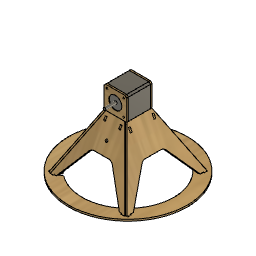
stepper stand v6 (Autodesk Fusion 360 design; units mm, degrees)
Autodesk Fusion 360 part; units mm, degrees
(part 1 of 2)
sketch "Sketch1" plane through (0, 0, 0) normal (0, 1, 0) x (1, 0, 0) in component "stepper"
  circle A0 centre (0, 0) radius 2.5
  circle A1 centre (0, 0) radius 12
  line L0 (21, 21) -> (-21, 21)
  line L1 (-21, 21) -> (-21, -21)
  line L2 (-21, -21) -> (21, -21)
  line L3 (21, -21) -> (21, 21)
  line L4 (21, 21) -> (-21, -21) construction
  line L5 (-21, 21) -> (21, -21) construction
  line L6 (-15.5, -15.5) -> (15.5, -15.5) construction
  line L7 (15.5, -15.5) -> (15.5, 15.5) construction
  line L8 (15.5, 15.5) -> (-15.5, 15.5) construction
  line L9 (-15.5, 15.5) -> (-15.5, -15.5) construction
  line L10 (-15.5, -15.5) -> (15.5, 15.5) construction
  line L11 (15.5, -15.5) -> (-15.5, 15.5) construction
  circle A2 centre (15.5, -15.5) radius 1.5
  circle A3 centre (-15.5, -15.5) radius 1.5
  circle A4 centre (-15.5, 15.5) radius 1.5
  circle A5 centre (15.5, 15.5) radius 1.5
  dimension "d1" = 5
  dimension "d2" = 24
  dimension "d3" = 42
  dimension "d4" = 42
  dimension "d5" = 31
  dimension "d6" = 31
  dimension "d7" = 3
  dimension "d8" = 3
  dimension "d9" = 3
  dimension "d10" = 3
  constraint coincident A0.centre A1.centre
  constraint concentric A0 A1
  constraint horizontal L0
  constraint perpendicular L0 L1
  constraint parallel L0 L2
  constraint parallel L1 L3
  constraint coincident L4 A0.centre
  constraint coincident L5 A0.centre
  constraint horizontal L6
  constraint perpendicular L6 L7
  constraint parallel L6 L8
  constraint parallel L7 L9
  constraint coincident L10 A0.centre
  constraint coincident L11 A0.centre
  constraint coincident L6.end L7.start
  constraint coincident L6.start L9.end
  constraint coincident L8.end L9.start
  constraint coincident L7.end L8.start
  measures "d1" diameter of A0
  measures "d2" diameter of A1
  measures "d3" distance of L1.end L2.end
  measures "d4" distance of L0.end L1.end
  measures "d5" distance of L7.end L8.end
  measures "d6" distance of L6.end L7.end
  measures "d7" diameter of A2
  measures "d8" diameter of A3
  measures "d9" diameter of A4
  measures "d10" diameter of A5
extrude "Extrude1" add sketch "Sketch1" against normal blind 41 from surface at 20.5 contours A0 | A1 | L0 L1 L2 L3 | A2 | A3 | A4 | A5 makes body 1 in component "stepper"
extrude "Extrude2" add sketch "Sketch1" against normal blind 2 from surface at -20.5 contours A0 | A1 bodies 1 in component "stepper"
extrude "Extrude3" add sketch "Sketch1" against normal blind 21 from surface at -22.5 contours A0 bodies 1 in component "stepper"
extrude "Extrude4" cut sketch "Sketch1" along normal blind 5 from surface at -20.5 contours A2 | A3 | A4 | A5 bodies 1 in component "stepper"
sketch "Sketch1 (2)" plane through (0, 0, 0) normal (0, 1, 0) x (1, 0, 0) in component "front plate"
  circle A0 centre (15.5, -15.5) radius 1.5
  circle A1 centre (15.5, 15.5) radius 1.5
  circle A2 centre (-15.5, -15.5) radius 1.5
  circle A3 centre (-15.5, 15.5) radius 1.5
  circle A4 centre (0, 0) radius 12
  line L0 (21, 21) -> (21, -21)
  line L1 (21, -21) -> (-21, -21)
  line L2 (-21, -21) -> (-21, 21)
  line L3 (-21, 21) -> (21, 21)
  line L4 (0, 21) -> (0, 121) construction
  line L5 (-142.4653, 121) -> (140, 121) construction
  line L6 (21, 21) -> (71.9525, 121)
  line L7 (21, 21) -> (155.3334, 21) construction
  line L8 (-21, 21) -> (-71.9525, 121)
  line L9 (13.9709, 71) -> (-46.4763, 71)
  line L10 (-17.633, 21) -> (-68.5856, 121)
  line L11 (17.633, 21) -> (68.5856, 121)
  line L12 (-21, 21) -> (-18.327, 22.362)
  line L13 (21, 21) -> (18.327, 22.362)
  line L14 (-25.2759, 36) -> (25.2759, 36)
  line L15 (68.5856, 121) -> (58.5856, 121)
  line L16 (58.5856, 121) -> (21.7954, 74.7728)
  arc A5 (13.9709, 71) -> (21.7954, 74.7728) centre (13.9709, 81) ccw
  line L17 (-68.5856, 121) -> (-58.5856, 121)
  line L18 (-58.5856, 121) -> (-21.7954, 74.7728)
  arc A6 (-21.7954, 74.7728) -> (-13.9709, 71) centre (-13.9709, 81) ccw
  line L19 (25.2759, 36) -> (27.9489, 34.638)
  line L20 (24.317, 27.51) -> (21.644, 28.8719)
  line L21 (-25.2759, 36) -> (-27.9489, 34.638)
  line L22 (-24.317, 27.51) -> (-21.644, 28.8719)
  line L23 (12.5, 21) -> (12.5, 36)
  line L24 (15.5, 21) -> (15.5, 36)
  line L25 (12.5, 28.5) -> (15.5, 28.5)
  line L26 (-12.5, 21) -> (-12.5, 36)
  line L27 (-15.5, 21) -> (-15.5, 36)
  line L28 (-12.5, 28.5) -> (-15.5, 28.5)
  dimension "d23" = 100
  dimension "d24" = 63
  dimension "d25" = 50
  dimension "d28" = 3
  dimension "d29" = 3
  dimension "d30" = 15
  dimension "d31" = 10
  dimension "d32" = 10
  dimension "d33" = 8
  dimension "d34" = 12.5
  dimension "d35" = 3
  constraint midpoint L3 L4.start
  constraint perpendicular L3 L4
  constraint perpendicular L4 L5
  constraint horizontal L7
  constraint coincident L0.start L3.end
  constraint coincident L5 L6.end
  constraint symmetric L4 L0.start L2.end
  constraint symmetric L4 L6.end L8.end
  constraint coincident L4.end L5
  constraint coincident L8 L9.end
  constraint horizontal L9
  constraint parallel L8 L10
  constraint coincident L3 L10.start
  constraint parallel L6 L11
  constraint coincident L3 L11.start
  constraint coincident L2.end L3.start
  constraint coincident L10 L12.end
  constraint perpendicular L10 L12
  constraint coincident L11 L13.end
  constraint perpendicular L11 L13
  constraint coincident L10 L14.start
  constraint coincident L11 L14.end
  constraint horizontal L14
  constraint coincident L5 L10.end
  constraint coincident L5 L11.end
  constraint coincident L5 L15.end
  constraint coincident L2.end L16
  constraint tangent L16 A5
  constraint tangent L9 A5
  constraint symmetric L4 L11.end L10.end
  constraint symmetric L4 L15.end L17.end
  constraint symmetric L4 L16.end L18.end
  constraint symmetric L4 L9.start A6.end
  constraint symmetric L4 A5 A6
  constraint coincident L6 L19.end
  constraint perpendicular L6 L19
  constraint coincident L6 L20.start
  constraint coincident L11 L20.end
  constraint perpendicular L11 L20
  constraint symmetric L4 L14.end L14.start
  constraint symmetric L4 L19.end L21.end
  constraint symmetric L4 L20.start L22.start
  constraint symmetric L4 L20.end L22.end
  constraint coincident L3 L23.start
  constraint coincident L14 L23.end
  constraint perpendicular L14 L23
  constraint coincident L3 L24.start
  constraint coincident L14 L24.end
  constraint perpendicular L14 L24
  constraint midpoint L23 L25.start
  constraint midpoint L24 L25.end
  constraint symmetric L4 L23.start L26.start
  constraint symmetric L4 L23.end L26.end
  constraint symmetric L4 L24.start L27.start
  constraint symmetric L4 L24.end L27.end
  constraint symmetric L4 L25.start L28.start
  constraint symmetric L4 L25.end L28.end
  measures "d23" distance of L4.start L4.end
  measures "d24" angle of L6 L7
  measures "d25" distance of L3 L9
  measures "d28" distance of L0.start L13.end
  measures "d29" distance of L2.end L12.end
  measures "d30" distance of L3 L14
  measures "d31" distance of L11.end L15.end
  measures "d32" radius of A5
  measures "d33" distance of L19 L20
  measures "d34" distance of L4 L23
  measures "d35" distance of L23 L24
extrude "Extrude1'" add sketch "Sketch1 (2)" against normal blind 3 from surface at -20.5 separate body contours L0 L1 L2 L3 | L3 L11 L14 L24 | L6 L11 L19 L20 | L3 L23 L24 L25 | L3 L14 L23 L26 | L3 L10 L14 L27 | L8 L10 L21 L22 | L3 L26 L27 L28 makes body 2 in component "front plate"
extrude "Extrude2'" add sketch "Sketch1 (2)" along normal blind 3 from surface at 20.5 separate body contours A0 | A1 | A2 | A3 | A4 | L0 L1 L2 L3 | L3 L11 L14 L24 | L6 L11 L19 L20 | L3 L23 L24 L25 | L3 L14 L23 L26 | L3 L10 L14 L27 | L8 L10 L21 L22 | L3 L26 L27 L28 makes body 3 in component "front plate"
sketch "Sketch1 (3)" plane through (0, 0, 0) normal (1, 0, 0) x (0, 1, 0) in component "side plate"
  line L0 (20.5, -21) -> (20.5, 21)
  line L1 (20.5, 21) -> (-20.5, 21)
  line L2 (-20.5, 21) -> (-20.5, -21)
  line L3 (-20.5, -21) -> (20.5, -21)
  line L4 (20.5, 21) -> (20.5, -21)
  line L5 (20.5, -21) -> (23.5, -21)
  line L6 (23.5, -21) -> (23.5, 21)
  line L7 (23.5, 21) -> (20.5, 21)
  line L8 (-20.5, -21) -> (-20.5, 21)
  line L9 (-20.5, 21) -> (-23.5, 21)
  line L10 (-23.5, 21) -> (-23.5, -21)
  line L11 (-23.5, -21) -> (-20.5, -21)
  line L12 (-20.5, -36) -> (-20.5, -28.5)
  line L13 (-20.5, -28.5) -> (-23.5, -28.5)
  line L14 (-23.5, -28.5) -> (-23.5, -36)
  line L15 (-23.5, -36) -> (-20.5, -36)
  line L16 (20.5, -28.5) -> (20.5, -36)
  line L17 (20.5, -36) -> (23.5, -36)
  line L18 (23.5, -36) -> (23.5, -28.5)
  line L19 (23.5, -28.5) -> (20.5, -28.5)
  line L20 (-165.7609, -120.8985) -> (170, -120.8985) construction
  line L21 (0, 0) -> (0, -121) construction
  line L22 (23.5, -21) -> (74.4008, -120.8985)
  line L23 (23.5, -21) -> (135.2326, -21) construction
  line L24 (-23.5, -21) -> (-74.4008, -120.8985)
  line L25 (-31.1429, -36) -> (31.1429, -36)
  line L26 (20.133, -21) -> (71.0338, -120.8985)
  line L27 (23.5, -28.5) -> (26.5338, -26.9542)
  line L28 (23.5, -36) -> (29.5676, -32.9084)
  line L29 (-20.133, -21) -> (-71.0338, -120.8985)
  line L30 (-23.5, -36) -> (-29.5676, -32.9084)
  line L31 (-23.5, -28.5) -> (-26.5338, -26.9542)
  line L32 (-20.5, 21) -> (-20.5, -21)
  line L33 (20.5, 21) -> (20.5, -21)
  line L34 (-20.5, -28.5) -> (-20.5, -21)
  line L35 (20.5, -28.5) -> (20.5, -21)
  point P0 (0, -121)
  dimension "d42" = 63
  dimension "d43" = 3
  constraint horizontal L20
  constraint coincident L21.start origin
  constraint coincident P0 L21.end
  constraint horizontal L23
  constraint coincident L5.end L6.start
  constraint coincident L20 L22.end
  constraint symmetric L21 L5.end L10.end
  constraint symmetric L21 L22.end L24.end
  constraint coincident L24 L25.start
  constraint coincident L22 L25.end
  constraint horizontal L25
  constraint collinear L17 L25
  constraint coincident L3 L26.start
  constraint coincident L20 L26.end
  constraint parallel L22 L26
  constraint coincident L18.end L19.start
  constraint coincident L22 L27.end
  constraint perpendicular L22 L27
  constraint coincident L17.end L18.start
  constraint coincident L22 L28.end
  constraint perpendicular L22 L28
  constraint symmetric L21 L26.start L29.start
  constraint symmetric L21 L26.end L29.end
  constraint symmetric L21 L18.end L13.end
  constraint symmetric L21 L27.end L31.end
  constraint symmetric L21 L17.end L14.end
  constraint symmetric L21 L28.end L30.end
  constraint coincident L12.end L13.start
  constraint coincident L2.end L3.start
  constraint coincident L16.start L19.end
  constraint coincident L0.start L3.end
  measures "d42" angle of L22 L23
  measures "d43" distance of L22 L26
extrude "Extrude1''" add sketch "Sketch1 (3)" along normal blind 3 from surface at 12.5 separate body contours L3 L12 L16 L25 L26 L29 L34 L35 | L22 L26 L27 L28 | L18 L26 L27 L28 | L16 L17 L18 L19 L25 | L25 L26 L28 | L14 L29 L30 L31 | L24 L29 L30 L31 | L12 L13 L14 L15 L25 | L25 L29 L30 makes body 4 in component "side plate"
mirror "Mirror1" about plane through (0, 0, 0) normal (1, 0, 0) of bodies 4 makes body 5 in component "side plate"
sketch "Sketch2" plane through (0, 0, 0) normal (0, 1, 0) x (1, 0, 0) in component "front face"
  line L0 (58.5856, 121) -> (21.7954, 74.7728)
  arc A0 (13.9709, 71) -> (21.7954, 74.7728) centre (13.9709, 81) ccw
  arc A1 (-21.7954, 74.7728) -> (-13.9709, 71) centre (-13.9709, 81) ccw
  line L1 (13.9709, 71) -> (-46.4763, 71)
  line L2 (-58.5856, 121) -> (-21.7954, 74.7728)
  line L3 (-68.5856, 121) -> (-58.5856, 121)
  line L4 (-17.633, 21) -> (-68.5856, 121)
  line L5 (-21, 21) -> (21, 21)
  line L6 (17.633, 21) -> (68.5856, 121)
  line L7 (68.5856, 121) -> (58.5856, 121)
  line L8 (68.5856, 121) -> (62.5856, 121)
  line L9 (62.5856, 121) -> (62.5856, 124)
  line L10 (62.5856, 124) -> (68.5856, 124)
  line L11 (68.5856, 124) -> (68.5856, 121)
  line L12 (0, 21) -> (0, 121)
  line L13 (-62.5856, 121) -> (-62.5856, 124)
  line L14 (-68.5856, 121) -> (-62.5856, 121)
  line L15 (-68.5856, 124) -> (-68.5856, 121)
  line L16 (-62.5856, 124) -> (-68.5856, 124)
  point P0 (-68.5856, 121)
  point P1 (-68.5856, 121)
  dimension "d53" = 6
  dimension "d54" = 3
  constraint horizontal L8
  constraint vertical L9
  constraint horizontal L10
  constraint vertical L11
  constraint coincident L6.end L7.start
  constraint symmetric L6.end L12 P1
  constraint symmetric L8.end L12 L13.start
  constraint symmetric L9.end L12 L13.end
  constraint symmetric L10.end L12 L15.start
  measures "d53" distance of L6.end L8.end
  measures "d54" distance of L6.end L10.end
extrude "Extrude1'''" add sketch "Sketch2" along normal blind -200 and the other way blind -200 separate body makes body 6 in component "front face"
ref_plane "WorkPlane1" through (-14, -28.0507, -29.9313) normal (0, -0.891007, 0.45399) x (0, -0.45399, -0.891007) in component "front face"
split "Split1" by plane through (-14, -28.0507, -29.9313) normal (0, -0.891007, 0.45399) bodies 6 makes body 7 at (34.6172, -99.3175, -54.3333) in component "front face"
sketch "Sketch3" plane through (0, -10.1618, 5.1777) normal (0, -0.891007, 0.45399) x (1, 0, 0) in component "front face"
  line L0 (68.5856, -141.6125) -> (17.633, -29.3799)
  line L1 (17.633, -29.3799) -> (-17.633, -29.3799)
  line L2 (-17.633, -29.3799) -> (-68.5856, -141.6125)
  line L3 (-62.5856, -141.6125) -> (-58.5856, -141.6125)
  line L4 (-58.5856, -141.6125) -> (-21.7954, -89.7306)
  ellipse E0 centre (-13.9709, -96.7195) end of major axis (-13.9709, -85.4962) minor radius 10 (-13.9709, -85.4962) -> (-21.7954, -89.7306) ccw
  line L5 (-13.9709, -85.4962) -> (13.9709, -85.4962)
  ellipse E1 centre (13.9709, -96.7195) end of major axis (13.9709, -85.4962) minor radius 10 (21.7954, -89.7306) -> (13.9709, -85.4962) ccw
  line L6 (21.7954, -89.7306) -> (58.5856, -141.6125)
  line L7 (58.5856, -141.6125) -> (62.5856, -141.6125)
  line L8 (-17.633, -29.3799) -> (-68.3511, -141.0961)
  line L9 (-68.3511, -141.0961) -> (-60.9204, -141.0961)
  line L10 (-60.9204, -141.0961) -> (-24.729, -90.0586)
  ellipse E2 centre (-13.9709, -96.7195) end of major axis (-13.7968, -84.6799) minor radius 12.8971 (-13.9966, -84.6784) -> (-24.729, -90.0586) ccw
  line L11 (-13.9966, -84.6784) -> (13.8126, -84.6784)
  ellipse E3 centre (13.9709, -96.7195) end of major axis (13.5291, -84.6836) minor radius 9.6471 (21.1526, -88.8241) -> (13.8126, -84.6784) ccw
  line L12 (21.1526, -88.8241) -> (58.5856, -141.6125)
  line L13 (58.5856, -141.6125) -> (68.5856, -141.6125)
  line L14 (68.5856, -141.6125) -> (17.633, -29.3799)
  line L15 (17.633, -29.3799) -> (-17.633, -29.3799)
  line L16 (-68.5856, -144.9795) -> (-62.5856, -144.9795)
  line L17 (-62.5856, -144.9795) -> (-62.5856, -141.6125)
  line L18 (62.5856, -141.6125) -> (62.5856, -144.9795)
  line L19 (62.5856, -144.9795) -> (68.5856, -144.9795)
  line L20 (68.5856, -144.9795) -> (68.5856, -141.6125)
  line L21 (-68.5856, -141.6125) -> (-68.5856, -144.9795)
  line L22 (-12.5, -42.745) -> (-12.5, -36.0625)
  line L23 (-12.5, -36.0625) -> (-15.5, -36.0625)
  line L24 (-15.5, -36.0625) -> (-15.5, -42.745)
  line L25 (-15.5, -42.745) -> (-12.5, -42.745)
  line L26 (12.5, -36.0625) -> (12.5, -42.745)
  line L27 (12.5, -42.745) -> (15.5, -42.745)
  line L28 (15.5, -42.745) -> (15.5, -36.0625)
  line L29 (15.5, -36.0625) -> (12.5, -36.0625)
  circle A0 centre (0, -65) radius 2.25
  dimension "d55" = 4.5
  constraint parallel L2 L8
  constraint parallel L3 L9
  constraint parallel L4 L10
  constraint concentric E0 E2
  constraint parallel L5 L11
  constraint concentric E1 E3
  constraint parallel L6 L12
  constraint parallel L7 L13
  constraint parallel L0 L14
  constraint parallel L1 L15
  constraint tangent L10 E2
  constraint tangent E2 L11
  constraint tangent E3 L12
  constraint tangent L11 E3
  measures "d55" diameter of A0
extrude "Extrude2''" add sketch "Sketch3" against normal blind 3 separate body makes body 8 in component "front face"
draft "Draft1" angle -63 neutral plane through (0, -10.1618, 5.1777) pull (0, -0.891007, 0.45399) 1 faces at (5.8777, -22.609, -21.454) on bodies 8 in component "front face"
ref_plane "WorkPlane2" through (14, 28.0507, -29.9313) normal (0, 0.891007, 0.45399) x (0, -0.45399, 0.891007) in component "front face"
split "Split2" by plane through (14, 28.0507, -29.9313) normal (0, 0.891007, 0.45399) bodies 6 makes body 9 at (34.6172, 99.3175, -54.3333) in component "front face"
sketch "Sketch4" plane through (0, 10.1618, 5.1777) normal (0, 0.891007, 0.45399) x (-1, 0, 0) in component "front face"
  line L0 (-62.5856, -141.6125) -> (-58.5856, -141.6125)
  line L1 (-58.5856, -141.6125) -> (-21.7954, -89.7306)
  ellipse E0 centre (-13.9709, -96.7195) end of major axis (-13.9709, -85.4962) minor radius 10 (-13.9709, -85.4962) -> (-21.7954, -89.7306) ccw
  line L2 (-13.9709, -85.4962) -> (13.9709, -85.4962)
  ellipse E1 centre (13.9709, -96.7195) end of major axis (13.9709, -85.4962) minor radius 10 (21.7954, -89.7306) -> (13.9709, -85.4962) ccw
  line L3 (21.7954, -89.7306) -> (58.5856, -141.6125)
  line L4 (58.5856, -141.6125) -> (62.5856, -141.6125)
  line L5 (62.5856, -141.6125) -> (62.5856, -144.9795)
  line L6 (62.5856, -144.9795) -> (68.5856, -144.9795)
  line L7 (68.5856, -144.9795) -> (68.5856, -141.6125)
  line L8 (68.5856, -141.6125) -> (17.633, -29.3799)
  line L9 (17.633, -29.3799) -> (-17.633, -29.3799)
  line L10 (-17.633, -29.3799) -> (-68.5856, -141.6125)
  line L11 (-68.5856, -141.6125) -> (-68.5856, -144.9795)
  line L12 (-68.5856, -144.9795) -> (-62.5856, -144.9795)
  line L13 (-62.5856, -144.9795) -> (-62.5856, -141.6125)
  line L14 (-17.633, -29.3799) -> (-68.5856, -141.6125)
  line L15 (-68.5856, -141.6125) -> (-68.5856, -144.9795)
  line L16 (-68.5856, -144.9795) -> (-62.5856, -144.9795)
  line L17 (-62.5856, -144.9795) -> (-62.5856, -141.6125)
  line L18 (-62.5856, -141.6125) -> (-58.5856, -141.6125)
  line L19 (-58.5856, -141.6125) -> (-21.7954, -89.7306)
  ellipse E2 centre (-13.9709, -96.7195) end of major axis (-13.9709, -85.4962) minor radius 10 (-13.9709, -85.4962) -> (-21.7954, -89.7306) ccw
  line L20 (-13.9709, -85.4962) -> (13.9709, -85.4962)
  ellipse E3 centre (13.9709, -96.7195) end of major axis (13.9709, -85.4962) minor radius 10 (21.7954, -89.7306) -> (13.9709, -85.4962) ccw
  line L21 (21.7954, -89.7306) -> (58.5856, -141.6125)
  line L22 (58.5856, -141.6125) -> (62.5856, -141.6125)
  line L23 (62.5856, -141.6125) -> (62.5856, -144.9795)
  line L24 (62.5856, -144.9795) -> (68.5856, -144.9795)
  line L25 (68.5856, -144.9795) -> (68.5856, -141.6125)
  line L26 (68.5856, -141.6125) -> (17.633, -29.3799)
  line L27 (17.633, -29.3799) -> (-17.633, -29.3799)
  line L28 (-12.5, -42.745) -> (-12.5, -36.0625)
  line L29 (-12.5, -36.0625) -> (-15.5, -36.0625)
  line L30 (-15.5, -36.0625) -> (-15.5, -42.745)
  line L31 (-15.5, -42.745) -> (-12.5, -42.745)
  line L32 (12.5, -36.0625) -> (12.5, -42.745)
  line L33 (12.5, -42.745) -> (15.5, -42.745)
  line L34 (15.5, -42.745) -> (15.5, -36.0625)
  line L35 (15.5, -36.0625) -> (12.5, -36.0625)
  line L36 (0, -29.3799) -> (0, -121.839) construction
  circle A0 centre (0, -70.4962) radius 5.5
  circle A1 centre (0, -55.4962) radius 3
  dimension "d63" = 0
  dimension "d64" = 11
  dimension "d65" = 15
  dimension "d66" = 6
  dimension "d67" = 30
  constraint midpoint L27 L36.start
  constraint perpendicular L9 L36
  constraint coincident L36 A0.centre
  constraint coincident L36 A1.centre
  measures "d64" diameter of A0
  measures "d65" distance of L20 A0.centre
  measures "d66" diameter of A1
  measures "d67" distance of L20 A1.centre
extrude "Extrude3'" add sketch "Sketch4" against normal blind 3 separate body makes body 10 in component "front face"
draft "Draft2" angle -63 neutral plane through (0, 10.1618, 5.1777) pull (0, 0.891007, 0.45399) 1 faces at (-5.8777, 22.609, -21.454) on bodies 10 in component "front face"
ref_plane "WorkPlane1" through (0, 0, -121) normal (0, 0, 1) x (1, 0, 0) in component "sides"
sketch "Sketch3 (2)" plane through (0, 0, 0) normal (1, 0, 0) x (0, 1, 0) in component "sides"
  line L0 (74.4525, -121) -> (23.5, -21)
  line L1 (-23.5, -21) -> (-74.4525, -121)
  line L2 (35.783, -121) -> (1.2339, -121)
  line L3 (-23.5, -21) -> (23.5, -21)
  line L4 (-62.4525, -121) -> (-22.4689, -74.4817)
  line L5 (0, -71) -> (-14.8852, -71)
  arc A0 (-14.8852, -71) -> (-22.4689, -74.4817) centre (-14.8852, -81) ccw
  line L6 (-62.4525, -121) -> (23.5, -21) construction
  line L7 (0, -21) -> (0, -121) construction
  line L8 (0, -21) -> (0, -121)
  line L9 (-62.4525, -121) -> (-74.4525, -121)
  line L10 (-74.4525, -121) -> (-68.4525, -121)
  line L11 (-68.4525, -121) -> (-68.4525, -124)
  line L12 (-68.4525, -124) -> (-74.4525, -124)
  line L13 (-74.4525, -124) -> (-74.4525, -121)
  line L14 (62.4525, -121) -> (22.4689, -74.4817)
  line L15 (62.4525, -121) -> (-23.5, -21) construction
  line L16 (74.4525, -124) -> (74.4525, -121)
  line L17 (74.4525, -121) -> (68.4525, -121)
  line L18 (68.4525, -121) -> (68.4525, -124)
  line L19 (62.4525, -121) -> (74.4525, -121)
  line L20 (68.4525, -124) -> (74.4525, -124)
  line L21 (0, -71) -> (14.8852, -71)
  arc A1 (22.4689, -74.4817) -> (14.8852, -71) centre (14.8852, -81) ccw
  point P0 (74.4525, -121)
  dimension "d73" = 12
  dimension "d74" = 50
  dimension "d75" = 10
  dimension "d109" = 6
  dimension "d110" = 3
  constraint coincident L1.start L3.start
  constraint coincident L0.end L3.end
  constraint horizontal L5
  constraint tangent L4 A0
  constraint tangent L5 A0
  constraint parallel L4 L6
  constraint midpoint L3 L7.start
  constraint perpendicular L2 L7
  constraint coincident L7 L5.start
  constraint coincident L1.end L9.end
  constraint horizontal L9
  constraint horizontal L10
  constraint vertical L11
  constraint horizontal L12
  constraint vertical L13
  constraint symmetric L1.end L7 P0
  constraint symmetric L4.start L7 L14.start
  constraint symmetric L4.end L7 L14.end
  constraint symmetric L5.end L7 L21.end
  constraint symmetric A0 L7 A1
  constraint symmetric L0.end L7 L1.start
  constraint symmetric L7 L5.start L21.start
  constraint symmetric L7 L1.end P0
  constraint symmetric L7 L10.end L17.end
  constraint symmetric L7 L11.end L18.end
  constraint symmetric L7 L12.end L16.start
  measures "d73" distance of L1.end L4.start
  measures "d74" distance of L3 L5
  measures "d75" radius of A0
  measures "d109" distance of L1.end L10.end
  measures "d110" distance of L1.end L12.end
extrude "Extrude1''''" add sketch "Sketch3 (2)" along normal blind 200 and the other way blind 200 separate body contours L0 L3 L8 L14 L17 L19 L21 A1 | L1 L3 L4 L5 A0 L8 L9 L10 makes body 11 in component "sides"
ref_plane "WorkPlane2" through (-26.133, -22, -31.074) normal (-0.891007, 0, 0.45399) x (-0.45399, 0, -0.891007) in component "sides"
ref_plane "WorkPlane3" through (26.133, -22, -31.074) normal (0.891007, 0, 0.45399) x (-0.45399, 0, 0.891007) in component "sides"
split "Split1'" by plane through (-26.133, -22, -31.074) normal (-0.891007, 0, 0.45399) bodies 11 makes body 12 at (-97.6508, 40.4842, -54.3333) in component "sides"
split "Split2'" by plane through (26.133, -22, -31.074) normal (0.891007, 0, 0.45399) bodies 11 makes body 13 at (97.6508, 40.4842, -54.3333) in component "sides"
sketch "Sketch4 (2)" plane through (-8.1771, 0, 4.1664) normal (-0.891007, 0, 0.45399) x (0, -1, 0) in component "sides"
  line L0 (-73.9525, -140.4776) -> (-73.9525, -143.8445)
  line L1 (-73.9525, -143.8445) -> (-67.9525, -143.8445)
  line L2 (-67.9525, -143.8445) -> (-67.9525, -140.4776)
  line L3 (-67.9525, -140.4776) -> (-61.9525, -140.4776)
  line L4 (61.9525, -140.4776) -> (67.9525, -140.4776)
  line L5 (67.9525, -140.4776) -> (67.9525, -143.8445)
  line L6 (67.9525, -143.8445) -> (73.9525, -143.8445)
  line L7 (73.9525, -143.8445) -> (73.9525, -140.4776)
  line L8 (-20.5, -43.5513) -> (-20.5, -35.5513)
  line L9 (-20.5, -35.5513) -> (-23.5, -35.5513)
  line L10 (-23.5, -35.5513) -> (-23.5, -43.5513)
  line L11 (-23.5, -43.5513) -> (-20.5, -43.5513)
  line L12 (20.5, -35.5513) -> (20.5, -43.5513)
  line L13 (20.5, -43.5513) -> (23.5, -43.5513)
  line L14 (23.5, -43.5513) -> (23.5, -35.5513)
  line L15 (23.5, -35.5513) -> (20.5, -35.5513)
  line L16 (0, -30.2449) -> (0, -86.3612) construction
  line L17 (-11.5, -34.3612) -> (11.5, -34.3612)
  line L18 (-8, -39.8612) -> (8, -39.8612)
  line L19 (8, -39.8612) -> (8, -57.8612)
  line L20 (8, -57.8612) -> (-8, -57.8612)
  line L21 (-8, -57.8612) -> (-8, -39.8612)
  circle A0 centre (11.5, -34.3612) radius 1.25
  circle A1 centre (-11.5, -34.3612) radius 1.25
  line L22 (-62.4525, -140.4776) -> (-22.4689, -88.2688)
  ellipse E0 centre (-14.8852, -95.5845) end of major axis (-14.8852, -84.3612) minor radius 10 (-14.8852, -84.3612) -> (-22.4689, -88.2688) ccw
  line L23 (-14.8852, -84.3612) -> (14.8852, -84.3612)
  ellipse E1 centre (14.8852, -95.5845) end of major axis (14.8852, -84.3612) minor radius 10 (22.4689, -88.2688) -> (14.8852, -84.3612) ccw
  line L24 (22.4689, -88.2688) -> (62.4525, -140.4776)
  line L25 (62.4525, -140.4776) -> (74.4525, -140.4776)
  line L26 (74.4525, -140.4776) -> (23.5, -28.2449)
  line L27 (23.5, -28.2449) -> (-23.5, -28.2449)
  line L28 (-23.5, -28.2449) -> (-74.4525, -140.4776)
  line L29 (-74.4525, -140.4776) -> (-62.4525, -140.4776)
  dimension "d97" = 11.5
  dimension "d98" = 11.5
  dimension "d102" = 16
  dimension "d103" = 18
  dimension "d104" = 5.5
  dimension "d105" = 2.5
  dimension "d106" = 2.5
  dimension "d111" = 6.1163
  constraint perpendicular L16 L17
  constraint horizontal L18
  constraint vertical L19
  constraint horizontal L20
  constraint vertical L21
  constraint symmetric L16 L19 L21
  constraint coincident L17.end A0.centre
  constraint coincident L17.start A1.centre
  measures "d97" distance of L16 L17.end
  measures "d98" distance of L16 L17.start
  measures "d102" distance of L18.start L18.end
  measures "d103" distance of L18.end L19.end
  measures "d104" distance of L17 L18
  measures "d105" diameter of A0
  measures "d106" diameter of A1
  measures "d111" distance of L17 L27
extrude "Extrude2'''" add sketch "Sketch4 (2)" against normal blind 3 separate body makes body 14 in component "sides"
sketch "Sketch5" plane through (8.1771, 0, 4.1664) normal (0.891007, 0, 0.45399) x (0, 1, 0) in component "sides"
  line L0 (-23, -28.2449) -> (-73.9525, -140.4776)
  line L1 (-73.9525, -140.4776) -> (-73.9525, -143.8445)
  line L2 (-73.9525, -143.8445) -> (-67.9525, -143.8445)
  line L3 (-67.9525, -143.8445) -> (-67.9525, -140.4776)
  line L4 (-67.9525, -140.4776) -> (-61.9525, -140.4776)
  line L5 (-61.9525, -140.4776) -> (-22.4714, -88.3181)
  ellipse E0 centre (-14.8502, -95.5845) end of major axis (-14.8502, -84.3612) minor radius 10 (-14.8502, -84.3612) -> (-22.4714, -88.3181) ccw
  line L6 (-14.8502, -84.3612) -> (14.8502, -84.3612)
  ellipse E1 centre (14.8502, -95.5845) end of major axis (14.8502, -84.3612) minor radius 10 (22.4714, -88.3181) -> (14.8502, -84.3612) ccw
  line L7 (22.4714, -88.3181) -> (61.9525, -140.4776)
  line L8 (61.9525, -140.4776) -> (67.9525, -140.4776)
  line L9 (67.9525, -140.4776) -> (67.9525, -143.8445)
  line L10 (67.9525, -143.8445) -> (73.9525, -143.8445)
  line L11 (73.9525, -143.8445) -> (73.9525, -140.4776)
  line L12 (73.9525, -140.4776) -> (23, -28.2449)
  line L13 (23, -28.2449) -> (-23, -28.2449)
  line L14 (-20.5, -43.5513) -> (-20.5, -35.5513)
  line L15 (-20.5, -35.5513) -> (-23.5, -35.5513)
  line L16 (-23.5, -35.5513) -> (-23.5, -43.5513)
  line L17 (-23.5, -43.5513) -> (-20.5, -43.5513)
  line L18 (20.5, -35.5513) -> (20.5, -43.5513)
  line L19 (20.5, -43.5513) -> (23.5, -43.5513)
  line L20 (23.5, -43.5513) -> (23.5, -35.5513)
  line L21 (23.5, -35.5513) -> (20.5, -35.5513)
  line L22 (62.4525, -140.4776) -> (74.4525, -140.4776)
  line L23 (74.4525, -140.4776) -> (23.5, -28.2449)
  line L24 (23.5, -28.2449) -> (-23.5, -28.2449)
  line L25 (-23.5, -28.2449) -> (-74.4525, -140.4776)
  line L26 (-74.4525, -140.4776) -> (-62.4525, -140.4776)
  line L27 (-62.4525, -140.4776) -> (-22.4689, -88.2688)
  ellipse E2 centre (-14.8852, -95.5845) end of major axis (-14.8852, -84.3612) minor radius 10 (-14.8852, -84.3612) -> (-22.4689, -88.2688) ccw
  line L28 (-14.8852, -84.3612) -> (14.8852, -84.3612)
  ellipse E3 centre (14.8852, -95.5845) end of major axis (14.8852, -84.3612) minor radius 10 (22.4689, -88.2688) -> (14.8852, -84.3612) ccw
  line L29 (22.4689, -88.2688) -> (62.4525, -140.4776)
  constraint tangent E0 L6
  constraint tangent L6 E1
  constraint tangent L5 E0
  constraint tangent E1 L7
extrude "Extrude3''" add sketch "Sketch5" against normal blind 3 separate body contours L0 L4 E0 L6 E1 L8 L12 L13 L22 L24 L26 L27 E2 L28 E3 L29 | L1 L2 L3 L26 | L9 L10 L11 L22 | L4 L5 E0 L27 E2 | E1 L7 L8 E3 L29 makes body 15 in component "sides"
ref_plane "WorkPlane1" through (0, 0, -121) normal (0, 0, 1) x (1, 0, 0) in component "Base"
sketch "Sketch1 (4)" plane through (0, 0, -121) normal (0, 0, 1) x (1, 0, 0) in component "Base"
  ellipse E0 centre (0, -36.9982) end of major axis (2.25, -36.9982) minor radius 1.0215
  line L0 (-15.5, -26.8946) -> (-12.5, -26.8946)
  line L1 (-12.5, -26.8946) -> (-12.5, -23.8608)
  line L2 (-12.5, -23.8608) -> (-15.5, -23.8608)
  line L3 (-15.5, -23.8608) -> (-15.5, -26.8946)
  line L4 (15.5, -23.8608) -> (12.5, -23.8608)
  line L5 (12.5, -23.8608) -> (12.5, -26.8946)
  line L6 (12.5, -26.8946) -> (15.5, -26.8946)
  line L7 (15.5, -26.8946) -> (15.5, -23.8608)
  line L8 (58.5856, -71.7795) -> (21.7954, -48.2256)
  ellipse E1 centre (13.9709, -51.3985) end of major axis (3.9709, -51.3985) minor radius 5.0953 (21.7954, -48.2256) -> (13.9709, -46.3033) ccw
  line L9 (13.9709, -46.3033) -> (-13.9709, -46.3033)
  ellipse E2 centre (-13.9709, -51.3985) end of major axis (-23.9709, -51.3985) minor radius 5.0953 (-13.9709, -46.3033) -> (-21.7954, -48.2256) ccw
  line L10 (-21.7954, -48.2256) -> (-58.5856, -71.7795)
  line L11 (-58.5856, -71.7795) -> (-62.5856, -71.7795)
  line L12 (-62.5856, -71.7795) -> (-62.5856, -73.3081)
  line L13 (-62.5856, -73.3081) -> (-68.5856, -73.3081)
  line L14 (-68.5856, -73.3081) -> (-68.5856, -71.7795)
  line L15 (-68.5856, -71.7795) -> (-20.306, -23.5)
  line L16 (-20.306, -23.5) -> (20.306, -23.5)
  line L17 (20.306, -23.5) -> (68.5856, -71.7795)
  line L18 (68.5856, -71.7795) -> (68.5856, -73.3081)
  line L19 (68.5856, -73.3081) -> (62.5856, -73.3081)
  line L20 (62.5856, -73.3081) -> (62.5856, -71.7795)
  line L21 (62.5856, -71.7795) -> (58.5856, -71.7795)
  line L22 (25.2759, -23.5) -> (25.2759, -20.5)
  line L23 (25.2759, -20.5) -> (21.644, -20.5)
  line L24 (21.644, -20.5) -> (21.644, -23.5)
  line L25 (21.644, -23.5) -> (25.2759, -23.5)
  line L26 (21.644, 23.5) -> (21.644, 20.5)
  line L27 (21.644, 20.5) -> (25.2759, 20.5)
  line L28 (25.2759, 20.5) -> (25.2759, 23.5)
  line L29 (25.2759, 23.5) -> (21.644, 23.5)
  line L30 (69.2795, 61.9525) -> (45.5996, 22.4714)
  ellipse E3 centre (48.8985, 14.8502) end of major axis (48.8985, 4.8502) minor radius 5.0953 (45.5996, 22.4714) -> (43.8033, 14.8502) ccw
  line L31 (43.8033, 14.8502) -> (43.8033, -14.8502)
  ellipse E4 centre (48.8985, -14.8502) end of major axis (48.8985, -24.8502) minor radius 5.0953 (43.8033, -14.8502) -> (45.5996, -22.4714) ccw
  line L32 (45.5996, -22.4714) -> (69.2795, -61.9525)
  line L33 (69.2795, -61.9525) -> (69.2795, -67.9525)
  line L34 (69.2795, -73.9525) -> (18.327, -23)
  line L35 (18.327, -23) -> (18.327, 23)
  line L36 (18.327, 23) -> (69.2795, 73.9525)
  line L37 (69.2795, 73.9525) -> (70.8081, 73.9525)
  line L38 (70.8081, 73.9525) -> (70.8081, 67.9525)
  line L39 (70.8081, 67.9525) -> (69.2795, 67.9525)
  line L40 (69.2795, 67.9525) -> (69.2795, 61.9525)
  line L41 (-15.5, 23.8608) -> (-12.5, 23.8608)
  line L42 (-12.5, 23.8608) -> (-12.5, 26.8946)
  line L43 (-12.5, 26.8946) -> (-15.5, 26.8946)
  line L44 (-15.5, 26.8946) -> (-15.5, 23.8608)
  line L45 (15.5, 26.8946) -> (12.5, 26.8946)
  line L46 (12.5, 26.8946) -> (12.5, 23.8608)
  line L47 (12.5, 23.8608) -> (15.5, 23.8608)
  line L48 (15.5, 23.8608) -> (15.5, 26.8946)
  ellipse E5 centre (0, 39.4934) end of major axis (-5.5, 39.4934) minor radius 2.4969
  ellipse E6 centre (0, 32.6835) end of major axis (-3, 32.6835) minor radius 1.362
  line L49 (-58.5856, 71.7795) -> (-21.7954, 48.2256)
  ellipse E7 centre (-13.9709, 51.3985) end of major axis (-3.9709, 51.3985) minor radius 5.0953 (-21.7954, 48.2256) -> (-13.9709, 46.3033) ccw
  line L50 (-13.9709, 46.3033) -> (13.9709, 46.3033)
  ellipse E8 centre (13.9709, 51.3985) end of major axis (23.9709, 51.3985) minor radius 5.0953 (13.9709, 46.3033) -> (21.7954, 48.2256) ccw
  line L51 (21.7954, 48.2256) -> (58.5856, 71.7795)
  line L52 (58.5856, 71.7795) -> (62.5856, 71.7795)
  line L53 (62.5856, 71.7795) -> (62.5856, 73.3081)
  line L54 (62.5856, 73.3081) -> (68.5856, 73.3081)
  line L55 (68.5856, 73.3081) -> (68.5856, 71.7795)
  line L56 (68.5856, 71.7795) -> (20.306, 23.5)
  line L57 (20.306, 23.5) -> (-20.306, 23.5)
  line L58 (-20.306, 23.5) -> (-68.5856, 71.7795)
  line L59 (-68.5856, 71.7795) -> (-68.5856, 73.3081)
  line L60 (-68.5856, 73.3081) -> (-62.5856, 73.3081)
  line L61 (-62.5856, 73.3081) -> (-62.5856, 71.7795)
  line L62 (-62.5856, 71.7795) -> (-58.5856, 71.7795)
  line L63 (-69.2795, 62.4525) -> (-69.2795, 67.9525)
  line L64 (-69.2795, 67.9525) -> (-70.8081, 67.9525)
  line L65 (-70.8081, 67.9525) -> (-70.8081, 73.9525)
  line L66 (-70.8081, 73.9525) -> (-69.2795, 73.9525)
  line L67 (-69.2795, -67.9525) -> (-69.2795, -62.4525)
  circle A0 centre (0, 0) radius 110
  circle A1 centre (0, 0) radius 85
  line L68 (73.4811, -67.9525) -> (73.4811, -73.9525)
  line L69 (73.4811, -73.9525) -> (70.8081, -73.9525)
  line L70 (70.8081, -73.9525) -> (70.8081, -67.9525)
  line L71 (70.8081, -67.9525) -> (73.4811, -67.9525)
  line L72 (68.5856, -75.9811) -> (62.5856, -75.9811)
  line L73 (62.5856, -75.9811) -> (62.5856, -73.3081)
  line L74 (62.5856, -73.3081) -> (68.5856, -73.3081)
  line L75 (68.5856, -73.3081) -> (68.5856, -75.9811)
  line L76 (69.2795, -73.9525) -> (68.5856, -73.9525)
  line L77 (62.5856, -71.7795) -> (62.5856, -70.7795)
  line L78 (62.5856, -70.7795) -> (69.2795, -70.7795)
  line L79 (69.2795, -70.7795) -> (69.2795, -67.9525)
  line L80 (0, 0) -> (155.8484, 0) construction
  line L81 (0, 0) -> (0, -125.3516) construction
  line L82 (69.2795, 73.9525) -> (68.5856, 73.9525)
  line L83 (62.5856, 71.7795) -> (62.5856, 70.7795)
  line L84 (62.5856, 70.7795) -> (69.2795, 70.7795)
  line L85 (69.2795, 70.7795) -> (69.2795, 67.9525)
  line L86 (-69.2795, 73.9525) -> (-68.5856, 73.9525)
  line L87 (-62.5856, 71.7795) -> (-62.5856, 70.7795)
  line L88 (-62.5856, 70.7795) -> (-69.2795, 70.7795)
  line L89 (-69.2795, 70.7795) -> (-69.2795, 67.9525)
  line L90 (-69.2795, -70.7795) -> (-69.2795, -67.9525)
  line L91 (-62.5856, -70.7795) -> (-69.2795, -70.7795)
  line L92 (-62.5856, -71.7795) -> (-62.5856, -70.7795)
  line L93 (-69.2795, -73.9525) -> (-68.5856, -73.9525)
  line L94 (73.4811, 73.9525) -> (73.4811, 67.9525)
  line L95 (73.4811, 67.9525) -> (70.8081, 67.9525)
  line L96 (70.8081, 67.9525) -> (70.8081, 73.9525)
  line L97 (70.8081, 73.9525) -> (73.4811, 73.9525)
  line L98 (62.5856, 75.9811) -> (68.5856, 75.9811)
  line L99 (68.5856, 75.9811) -> (68.5856, 73.3081)
  line L100 (68.5856, 73.3081) -> (62.5856, 73.3081)
  line L101 (62.5856, 73.3081) -> (62.5856, 75.9811)
  line L102 (-68.5856, 75.9811) -> (-62.5856, 75.9811)
  line L103 (-62.5856, 75.9811) -> (-62.5856, 73.3081)
  line L104 (-62.5856, 73.3081) -> (-68.5856, 73.3081)
  line L105 (-68.5856, 73.3081) -> (-68.5856, 75.9811)
  line L106 (-73.4811, 67.9525) -> (-73.4811, 73.9525)
  line L107 (-73.4811, 73.9525) -> (-70.8081, 73.9525)
  line L108 (-70.8081, 73.9525) -> (-70.8081, 67.9525)
  line L109 (-70.8081, 67.9525) -> (-73.4811, 67.9525)
  line L110 (-73.4811, -73.9525) -> (-73.4811, -67.9525)
  line L111 (-73.4811, -67.9525) -> (-70.8081, -67.9525)
  line L112 (-70.8081, -67.9525) -> (-70.8081, -73.9525)
  line L113 (-70.8081, -73.9525) -> (-73.4811, -73.9525)
  line L114 (-62.5856, -75.9811) -> (-68.5856, -75.9811)
  line L115 (-68.5856, -75.9811) -> (-68.5856, -73.3081)
  line L116 (-68.5856, -73.3081) -> (-62.5856, -73.3081)
  line L117 (-62.5856, -73.3081) -> (-62.5856, -75.9811)
  line L118 (69.2795, -67.9525) -> (70.8081, -67.9525)
  line L119 (70.8081, -67.9525) -> (70.8081, -73.9525)
  line L120 (70.8081, -73.9525) -> (69.2795, -73.9525)
  line L121 (-69.2795, -73.9525) -> (-70.8081, -73.9525)
  line L122 (-70.8081, -73.9525) -> (-70.8081, -67.9525)
  line L123 (-70.8081, -67.9525) -> (-69.2795, -67.9525)
  line L124 (-69.2795, -62.4525) -> (-45.5773, -22.4689)
  ellipse E9 centre (-48.8985, -14.8852) end of major axis (-48.8985, -4.8852) minor radius 5.0953 (-45.5773, -22.4689) -> (-43.8033, -14.8852) ccw
  line L125 (-43.8033, -14.8852) -> (-43.8033, 14.8852)
  ellipse E10 centre (-48.8985, 14.8852) end of major axis (-48.8985, 24.8852) minor radius 5.0953 (-43.8033, 14.8852) -> (-45.5773, 22.4689) ccw
  line L126 (-45.5773, 22.4689) -> (-69.2795, 62.4525)
  line L127 (-69.2795, 73.9525) -> (-69.2795, 74.4525)
  line L128 (-69.2795, 74.4525) -> (-18.327, 23.5)
  line L129 (-18.327, 23.5) -> (-18.327, -23.5)
  line L130 (-18.327, -23.5) -> (-69.2795, -74.4525)
  line L131 (-69.2795, -74.4525) -> (-69.2795, -73.9525)
  line L132 (-31.7725, 8) -> (-31.7725, -8)
  line L133 (-31.7725, -8) -> (-23.6007, -8)
  line L134 (-23.6007, -8) -> (-23.6007, 8)
  line L135 (-23.6007, 8) -> (-31.7725, 8)
  line L136 (-25.2759, 23.5) -> (-25.2759, 20.5)
  line L137 (-25.2759, 20.5) -> (-21.644, 20.5)
  line L138 (-21.644, 20.5) -> (-21.644, 23.5)
  line L139 (-21.644, 23.5) -> (-25.2759, 23.5)
  ellipse E11 centre (-21.1037, 11.5) end of major axis (-21.1037, 10.25) minor radius 0.5675
  ellipse E12 centre (-21.1037, -11.5) end of major axis (-21.1037, -12.75) minor radius 0.5675
  line L140 (-21.644, -23.5) -> (-21.644, -20.5)
  line L141 (-21.644, -20.5) -> (-25.2759, -20.5)
  line L142 (-25.2759, -20.5) -> (-25.2759, -23.5)
  line L143 (-25.2759, -23.5) -> (-21.644, -23.5)
  dimension "d90" = 220
  dimension "d91" = 170
  dimension "d92" = 1
  constraint coincident A0.centre A1.centre
  constraint concentric A0 A1
  constraint coincident L20.end L21.start
  constraint coincident L34.start L76.start
  constraint coincident L75 L76.end
  constraint perpendicular L75 L76
  constraint perpendicular L21 L77
  constraint perpendicular L33 L78
  constraint coincident L33.end L79.end
  constraint perpendicular L46 L80
  constraint perpendicular L80 L81
  constraint symmetric L20.end L80 L52.end
  constraint symmetric L34.start L80 L36.end
  constraint symmetric L76.end L80 L82.end
  constraint symmetric L77.end L80 L83.end
  constraint symmetric L78.end L80 L84.end
  constraint symmetric L33.end L80 L39.end
  constraint symmetric L20.end L81 L11.end
  constraint symmetric L34.start L81 L93.start
  constraint symmetric L76.end L81 L93.end
  constraint symmetric L77.end L81 L91.start
  constraint symmetric L78.end L81 L90.start
  constraint symmetric L33.end L81 L67.start
  constraint symmetric L81 L36.end L66.end
  constraint symmetric L81 L82.end L86.end
  constraint symmetric L81 L52.end L61.end
  constraint symmetric L81 L83.end L87.end
  constraint symmetric L81 L84.end L88.end
  constraint symmetric L81 L39.end L63.end
  measures "d90" diameter of A0
  measures "d91" diameter of A1
  measures "d92" distance of L20.end L77.end
extrude "Extrude1'''''" add sketch "Sketch1 (4)" against normal blind 3 separate body contours L17 L32 L33 A1 L78 L79 | L18 L34 L75 L76 | L15 L67 A1 L90 L91 L124 | L17 L18 L34 L70 L78 L79 L118 L119 L120 | L14 L15 L90 L91 L93 L112 L115 L121 L122 L123 L130 | L58 L63 A1 L88 L89 L126 | L49 L62 A1 L87 L88 L128 | L58 A1 L88 L128 | L93 L115 L130 | L30 L40 L56 A1 L84 L85 | L36 L51 L52 A1 L83 L84 | L36 L56 A1 L84 | L93 L130 L131 | L86 L127 L128 | A0 makes body 16 in component "Base"
chamfer "Chamfer1" distance 3 angle 45 2 edges at (21, 0, 21) (-21, 0, 21) on bodies 1 in component "stepper"
chamfer "Chamfer1'" distance 3 angle 45 4 edges at (21, -22, 21) (-21, -22, 21) (21, 22, 21) (-21, 22, 21) on bodies 2 3 in component "front plate"
sketch "front_stepper" plane through (0, -23.5, 0) normal (0, -1, 0) x (1, 0, 0) in component "front plate"
  line L0 (-18, 21) -> (-21, 18)
  line L1 (-21, 18) -> (-21, -21)
  line L2 (-21, -21) -> (-17.633, -21)
  line L3 (-17.633, -21) -> (-21.644, -28.8719)
  line L4 (-21.644, -28.8719) -> (-24.317, -27.51)
  line L5 (-24.317, -27.51) -> (-27.9489, -34.638)
  line L6 (-27.9489, -34.638) -> (-25.2759, -36)
  line L7 (-25.2759, -36) -> (-15.5, -36)
  line L8 (-15.5, -36) -> (-15.5, -28.5)
  line L9 (-15.5, -28.5) -> (-12.5, -28.5)
  line L10 (-12.5, -28.5) -> (-12.5, -36)
  line L11 (-12.5, -36) -> (12.5, -36)
  line L12 (12.5, -36) -> (12.5, -28.5)
  line L13 (12.5, -28.5) -> (15.5, -28.5)
  line L14 (15.5, -28.5) -> (15.5, -36)
  line L15 (15.5, -36) -> (25.2759, -36)
  line L16 (25.2759, -36) -> (27.9489, -34.638)
  line L17 (27.9489, -34.638) -> (24.317, -27.51)
  line L18 (24.317, -27.51) -> (21.644, -28.8719)
  line L19 (21.644, -28.8719) -> (17.633, -21)
  line L20 (17.633, -21) -> (21, -21)
  line L21 (21, -21) -> (21, 18)
  line L22 (21, 18) -> (18, 21)
  line L23 (18, 21) -> (-18, 21)
  circle A0 centre (0, 0) radius 12
  circle A1 centre (-15.5, -15.5) radius 1.5
  circle A2 centre (15.5, 15.5) radius 1.5
  circle A3 centre (15.5, -15.5) radius 1.5
  circle A4 centre (-15.5, 15.5) radius 1.5
sketch "rear_stepper" plane through (0, 23.5, 0) normal (0, 1, 0) x (-1, 0, 0) in component "front plate"
  line L0 (21, 18) -> (18, 21)
  line L1 (18, 21) -> (-18, 21)
  line L2 (-18, 21) -> (-21, 18)
  line L3 (-21, 18) -> (-21, -21)
  line L4 (-21, -21) -> (-17.633, -21)
  line L5 (-17.633, -21) -> (-21.644, -28.8719)
  line L6 (-21.644, -28.8719) -> (-24.317, -27.51)
  line L7 (-24.317, -27.51) -> (-27.9489, -34.638)
  line L8 (-27.9489, -34.638) -> (-25.2759, -36)
  line L9 (-25.2759, -36) -> (-15.5, -36)
  line L10 (-15.5, -36) -> (-15.5, -28.5)
  line L11 (-15.5, -28.5) -> (-12.5, -28.5)
  line L12 (-12.5, -28.5) -> (-12.5, -36)
  line L13 (-12.5, -36) -> (12.5, -36)
  line L14 (12.5, -36) -> (12.5, -28.5)
  line L15 (12.5, -28.5) -> (15.5, -28.5)
  line L16 (15.5, -28.5) -> (15.5, -36)
  line L17 (15.5, -36) -> (25.2759, -36)
  line L18 (25.2759, -36) -> (27.9489, -34.638)
  line L19 (27.9489, -34.638) -> (24.317, -27.51)
  line L20 (24.317, -27.51) -> (21.644, -28.8719)
  line L21 (21.644, -28.8719) -> (17.633, -21)
  line L22 (17.633, -21) -> (21, -21)
  line L23 (21, -21) -> (21, 18)
sketch "stepper_support" plane through (-12.5, 0, 0) normal (1, 0, 0) x (0, 1, 0) in component "side plate"
  line L0 (20.133, -21) -> (-20.133, -21)
  line L1 (-20.5, -28.5) -> (-23.5, -28.5)
  line L2 (-23.5, -28.5) -> (-26.5338, -26.9542)
  line L3 (-26.5338, -26.9542) -> (-29.5676, -32.9084)
  line L4 (-29.5676, -32.9084) -> (-26.8946, -34.2704)
  line L5 (-20.133, -21) -> (-20.5, -21.7202)
  line L6 (-27.7759, -36) -> (27.7759, -36)
  line L7 (27.7759, -36) -> (26.8946, -34.2704)
  line L8 (26.8946, -34.2704) -> (29.5676, -32.9084)
  line L9 (29.5676, -32.9084) -> (26.5338, -26.9542)
  line L10 (26.5338, -26.9542) -> (23.5, -28.5)
  line L11 (23.5, -28.5) -> (20.5, -28.5)
  line L12 (20.5, -28.5) -> (20.5, -21.7202)
  line L13 (20.5, -21.7202) -> (20.133, -21)
  line L14 (-20.5, -21.7202) -> (-20.5, -28.5)
  line L15 (-26.8946, -34.2704) -> (-27.7759, -36)
sketch "left_face" plane through (-8.1771, 0, 4.1664) normal (-0.891007, 0, 0.45399) x (0, -1, 0) in component "sides"
  line L0 (62.4525, -140.4776) -> (67.9525, -140.4776)
  line L1 (67.9525, -140.4776) -> (67.9525, -143.8445)
  line L2 (67.9525, -143.8445) -> (73.9525, -143.8445)
  line L3 (73.9525, -143.8445) -> (73.9525, -140.4776)
  line L4 (-73.9525, -140.4776) -> (-73.9525, -143.8445)
  line L5 (-73.9525, -143.8445) -> (-67.9525, -143.8445)
  line L6 (-67.9525, -143.8445) -> (-67.9525, -140.4776)
  line L7 (-67.9525, -140.4776) -> (-62.4525, -140.4776)
  line L8 (22.4689, -88.2688) -> (62.4525, -140.4776)
  line L9 (73.9525, -140.4776) -> (74.4525, -140.4776)
  line L10 (74.4525, -140.4776) -> (23.5, -28.2449)
  line L11 (23.5, -28.2449) -> (-23.5, -28.2449)
  line L12 (-23.5, -28.2449) -> (-74.4525, -140.4776)
  line L13 (-74.4525, -140.4776) -> (-73.9525, -140.4776)
  line L14 (-62.4525, -140.4776) -> (-22.4689, -88.2688)
  ellipse E0 centre (-14.8852, -95.5845) end of major axis (-14.8852, -84.3612) minor radius 10 (-14.8852, -84.3612) -> (-22.4689, -88.2688) ccw
  line L15 (-14.8852, -84.3612) -> (14.8852, -84.3612)
  ellipse E1 centre (14.8852, -95.5845) end of major axis (14.8852, -84.3612) minor radius 10 (22.4689, -88.2688) -> (14.8852, -84.3612) ccw
  line L16 (8, -57.8612) -> (-8, -57.8612)
  line L17 (-8, -57.8612) -> (-8, -39.8612)
  line L18 (-8, -39.8612) -> (8, -39.8612)
  line L19 (8, -39.8612) -> (8, -57.8612)
  line L20 (-20.5, -43.5513) -> (-23.5, -43.5513)
  line L21 (-23.5, -43.5513) -> (-23.5, -35.5513)
  line L22 (-23.5, -35.5513) -> (-20.5, -35.5513)
  line L23 (-20.5, -35.5513) -> (-20.5, -43.5513)
  circle A0 centre (-11.5, -34.3612) radius 1.25
  circle A1 centre (11.5, -34.3612) radius 1.25
  line L24 (20.5, -35.5513) -> (23.5, -35.5513)
  line L25 (23.5, -35.5513) -> (23.5, -43.5513)
  line L26 (23.5, -43.5513) -> (20.5, -43.5513)
  line L27 (20.5, -43.5513) -> (20.5, -35.5513)
sketch "front_face" plane through (0, -10.1618, 5.1777) normal (0, -0.891007, 0.45399) x (1, 0, 0) in component "front face"
  circle A0 centre (0, -65) radius 2.25
  line L0 (-12.5, -42.745) -> (-15.5, -42.745)
  line L1 (-15.5, -42.745) -> (-15.5, -36.0625)
  line L2 (-15.5, -36.0625) -> (-12.5, -36.0625)
  line L3 (-12.5, -36.0625) -> (-12.5, -42.745)
  line L4 (12.5, -36.0625) -> (15.5, -36.0625)
  line L5 (15.5, -36.0625) -> (15.5, -42.745)
  line L6 (15.5, -42.745) -> (12.5, -42.745)
  line L7 (12.5, -42.745) -> (12.5, -36.0625)
  line L8 (21.7954, -89.7306) -> (58.5856, -141.6125)
  line L9 (58.5856, -141.6125) -> (62.5856, -141.6125)
  line L10 (62.5856, -141.6125) -> (62.5856, -144.9795)
  line L11 (62.5856, -144.9795) -> (68.5856, -144.9795)
  line L12 (68.5856, -144.9795) -> (68.5856, -141.6125)
  line L13 (68.5856, -141.6125) -> (17.633, -29.3799)
  line L14 (17.633, -29.3799) -> (-17.633, -29.3799)
  line L15 (-17.633, -29.3799) -> (-68.5856, -141.6125)
  line L16 (-68.5856, -141.6125) -> (-68.5856, -144.9795)
  line L17 (-68.5856, -144.9795) -> (-62.5856, -144.9795)
  line L18 (-62.5856, -144.9795) -> (-62.5856, -141.6125)
  line L19 (-62.5856, -141.6125) -> (-58.5856, -141.6125)
  line L20 (-58.5856, -141.6125) -> (-21.7954, -89.7306)
  ellipse E0 centre (-13.9709, -96.7195) end of major axis (-13.9709, -85.4962) minor radius 10 (-13.9709, -85.4962) -> (-21.7954, -89.7306) ccw
  line L21 (-13.9709, -85.4962) -> (13.9709, -85.4962)
  ellipse E1 centre (13.9709, -96.7195) end of major axis (13.9709, -85.4962) minor radius 10 (21.7954, -89.7306) -> (13.9709, -85.4962) ccw
sketch "rear_face" plane through (0, 10.1618, 5.1777) normal (0, 0.891007, 0.45399) x (-1, 0, 0) in component "front face"
  line L0 (12.5, -36.0625) -> (15.5, -36.0625)
  line L1 (15.5, -36.0625) -> (15.5, -42.745)
  line L2 (15.5, -42.745) -> (12.5, -42.745)
  line L3 (12.5, -42.745) -> (12.5, -36.0625)
  line L4 (-12.5, -42.745) -> (-15.5, -42.745)
  line L5 (-15.5, -42.745) -> (-15.5, -36.0625)
  line L6 (-15.5, -36.0625) -> (-12.5, -36.0625)
  line L7 (-12.5, -36.0625) -> (-12.5, -42.745)
  circle A0 centre (0, -70.4962) radius 5.5
  circle A1 centre (0, -55.4962) radius 3
  line L8 (21.7954, -89.7306) -> (58.5856, -141.6125)
  line L9 (58.5856, -141.6125) -> (62.5856, -141.6125)
  line L10 (62.5856, -141.6125) -> (62.5856, -144.9795)
  line L11 (62.5856, -144.9795) -> (68.5856, -144.9795)
  line L12 (68.5856, -144.9795) -> (68.5856, -141.6125)
  line L13 (68.5856, -141.6125) -> (17.633, -29.3799)
  line L14 (17.633, -29.3799) -> (-17.633, -29.3799)
  line L15 (-17.633, -29.3799) -> (-68.5856, -141.6125)
  line L16 (-68.5856, -141.6125) -> (-68.5856, -144.9795)
  line L17 (-68.5856, -144.9795) -> (-62.5856, -144.9795)
  line L18 (-62.5856, -144.9795) -> (-62.5856, -141.6125)
  line L19 (-62.5856, -141.6125) -> (-58.5856, -141.6125)
  line L20 (-58.5856, -141.6125) -> (-21.7954, -89.7306)
  ellipse E0 centre (-13.9709, -96.7195) end of major axis (-13.9709, -85.4962) minor radius 10 (-13.9709, -85.4962) -> (-21.7954, -89.7306) ccw
  line L21 (-13.9709, -85.4962) -> (13.9709, -85.4962)
  ellipse E1 centre (13.9709, -96.7195) end of major axis (13.9709, -85.4962) minor radius 10 (21.7954, -89.7306) -> (13.9709, -85.4962) ccw